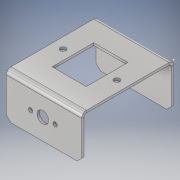
# Autodesk Inventor part: fc17-036
Saved by Autodesk Inventor 2017.1 (Build 211199000, 199)
## iProperties
Category: Controls
Company: Autodesk Inc.
Created: 2016-12-15
Part Number: fc17-036
Material: Aluminum 6061
Document SubType Name: Sheet Metal
Designer: Autodesk Inc.
Density: 2.7 g/cm^3
Sheet Metal Rule: Default
Appearance: Aluminum - Polished
Catalog Web Link: http://files.andymark.com/Camera-Pan-Tilt-Assembly.pdf
Vendor: ebm papst
Author: Autodesk Inc.
Keywords: FIRSTChoice
Autodesk Inventor part; units mm, degrees
ref_plane "YZ Plane" through (0, 0, 0) normal (1, 0, 0) x (0, 1, 0)
ref_plane "XZ Plane" through (0, 0, 0) normal (0, 1, 0) x (-1, 0, 0)
ref_plane "XY Plane" through (0, 0, 0) normal (0, 0, 1) x (1, 0, 0)
sketch "Sketch1" plane through (0, 0, 0) normal (0, 1, 0) x (-1, 0, 0)
  line L0 (0, 0) -> (52.324, 0)
  line L1 (52.324, 0) -> (52.324, -63.881)
  line L2 (52.324, -63.881) -> (0, -63.881)
  line L3 (0, -63.881) -> (0, 0)
  dimension "d0" = 52.324
  dimension "d1" = 63.881
  measures "d0" distance of L1.end L2.end
  measures "d1" distance of L0.end L1.end
extrude "Plate1" add sketch "Sketch1" against normal blind 1.6281
sketch "Sketch2" plane through (-52.324, 0, -1.6281) normal (0, 0, 1) x (1, 0, 0)
  line L0 (52.324, 0) -> (0, 0)
  line L1 (0, 0) -> (0, -30.48)
  line L2 (0, -30.48) -> (52.324, -30.48)
  line L3 (52.324, -30.48) -> (52.324, 0)
  constraints: 6 end point, 1 horizontal, 1 perpendicular, 1 vertical
edge flange "Flange1" height 30.48 angle 90 thickness 1.6281 bend radius 1.6281 thickness toward (0, 0, 1) relief straight relief width 1.6281 relief depth 0.8141 corner gap 1.6281 corner form 0 edges at (-26.162, -1.6281, 0) (-26.162, -1.6281, -63.881) wall of the first edge with corners at (0, 0, -1.6281) (-52.324, 0, -1.6281) (-52.324, -30.48, -1.6281) (0, -30.48, -1.6281)
bend "Bend1"
corner "Corner1"
sketch "Sketch3" plane through (0, 0, 0) normal (0, 1, 0) x (1, 0, 0)
  line L0 (-14.3002, 17.4752) -> (-38.0238, 17.4752)
  line L1 (-38.0238, 17.4752) -> (-38.0238, 46.4058)
  line L2 (-38.0238, 46.4058) -> (-14.3002, 46.4058)
  line L3 (-14.3002, 46.4058) -> (-14.3002, 17.4752)
  line L4 (0, 0) -> (-52.324, 0) projected
  line L5 (-52.324, 3.2563) -> (-52.324, 60.6247) projected
  dimension "d13" = 17.4752
  dimension "d14" = 46.4058
  dimension "d15" = 14.3002
  dimension "d16" = 38.0238
  constraints: 8 end point, 2 parallel, 1 horizontal, 1 perpendicular
  measures "d13" distance between parallel lines of L0 L4
  measures "d14" distance between parallel lines of L2 L4
  measures "d15" distance between parallel lines of L1 L5
  measures "d16" distance between parallel lines of L3 L5
extrude "Cut1" cut sketch "Sketch3" against normal blind 1.6281
sketch "Sketch4" plane through (0, 0, 0) normal (0, 1, 0) x (1, 0, 0)
  line L0 (-52.324, 3.2563) -> (-52.324, 60.6247) projected
  point P0 (0, 0)
  point P1 (-44.831, 31.9405)
  point P2 (-7.493, 31.9405)
  point P3 (-52.324, 31.9405)
  dimension "d19" = 7.493
  dimension "d20" = 44.831
  constraints: 2 horizontal alignment, 1 midpoint
  measures "d19" distance from line of point (-44.831, 31.941) L0
  measures "d20" distance from line of point (-7.493, 31.941) L0
hole "Hole1" at (-44.831, 0, -31.9405) at (-7.493, 0, -31.9405) direction (0, -1, 0) diameter 3.8862 end up to surface
sketch "Sketch5" plane through (-52.324, -30.48, 0) normal (0, 0, 1) x (1, 0, 0)
  line L0 (0, 30.48) -> (52.324, 30.48) projected
  line L1 (0, 0) -> (0, 27.2237) projected
  point P0 (16.891, 14.4526)
  point P1 (25.4, 14.4526)
  point P2 (33.909, 14.4526)
  dimension "d28" = 16.0274
  dimension "d29" = 16.891
  dimension "d30" = 25.4
  dimension "d31" = 33.909
  constraints: 2 horizontal alignment
  measures "d28" distance from line of point (16.891, 14.453) L0
  measures "d29" distance from line of point (16.891, 14.453) L1
  measures "d30" distance from line of point (25.4, 14.453) L1
  measures "d31" distance from line of point (33.909, 14.453) L1
hole "Hole2" at (-35.433, -16.0274, 0) at (-18.415, -16.0274, 0) direction (0, 0, -1) diameter 2.9464 end up to surface
hole "Hole3" at (-26.924, -16.0274, 0) direction (0, 0, -1) diameter 8.001 end up to surface
sketch "Sketch6" plane through (0, -30.48, -63.881) normal (0, 0, -1) x (-1, 0, 0)
  point P0 (0, 30.48)
sketch "Sketch7" plane through (0, -30.48, -63.881) normal (0, 0, -1) x (-1, 0, 0)
  circle A0 centre (26.924, 14.4526) radius 4.0005 projected
  point P0 (0, 30.48)
  constraints: 1 coincident
hole "Hole4" at (-26.924, -16.0274, -63.881) direction (0, 0, 1) diameter 4.318 end up to surface
chamfer "Corner Chamfer1" distance 3.175 angle 45 4 edges at (0, -30.48, -0.8141) (-52.324, -30.48, -0.8141) (0, -30.48, -63.0669) (-52.324, -30.48, -63.0669)
equation "\"d17\" = Thickness"
equation "\"d26\" = Thickness"
equation "\"d37\" = Thickness"
equation "\"d44\" = Thickness"
equation "\"d51\" = Thickness"
equation "\"d3\" = BendReliefWidth"
equation "\"d4\" = BendReliefDepth"
equation "\"d5\" = MinimumRemnant"
equation "\"d6\" = BendRadius"
equation "\"d9\" = BendRadius"
equation "\"d10\" = CornerReliefSize"
equation "\"d11\" = GapSize"
equation "\"d12\" = JacobiRadiusSize"
equation "\"BendRadius\" = Thickness"
equation "\"BendReliefWidth\" = Thickness"
equation "\"BendReliefDepth\" = 0.5 * Thickness"
equation "\"CornerReliefSize\" = 4 * Thickness"
equation "\"MinimumRemnant\" = 2 * Thickness"
equation "\"TransitionRadius\" = BendRadius"
equation "\"JacobiRadiusSize\" = BendRadius"
equation "\"GapSize\" = Thickness"
equation "\"d2\" = BendRadius"
equation "\"Thickness\" = 1.62814"
body "Solid1"
